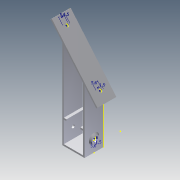
# Autodesk Inventor part: carousel_mount_bracket
Saved by Autodesk Inventor 2011 (Build 150239000, 239)
## iProperties
Created: 2012-12-04
Part Number: carousel_mount_bracket
Document SubType Name: Modeling
Designer: Administrator
Density: 1 g/cm^3
Author: Administrator
Autodesk Inventor part; units mm, degrees
ref_plane "YZ Plane" through (0, 0, 0) normal (1, 0, 0) x (0, 1, 0)
ref_plane "XZ Plane" through (0, 0, 0) normal (0, 1, 0) x (-1, 0, 0)
sketch "Sketch1" plane through (0, 0, 0) normal (0, 0, 1) x (1, 0, 0)
  line L0 (-12.4, 10.5) -> (12.4, 10.5)
  line L1 (12.4, 10.5) -> (12.4, -10.5)
  line L2 (12.4, -10.5) -> (-12.4, -10.5)
  line L3 (-12.4, -10.5) -> (-12.4, 10.5)
  point P0 (0, 0)
  point P1 (-12.4, 0)
  point P2 (0, 10.5)
  dimension "d0" = 24.8
  dimension "d1" = 21
  constraints: 8 end point, 2 midpoint, 2 parallel, 1 horizontal, 1 horizontal alignment, 1 perpendicular, 1 vertical alignment
  measures "d0" distance of L0.start L0.end
  measures "d1" distance between parallel lines of L2 L0
extrude "Extrusion1" add sketch "Sketch1" along normal blind 1.75
ref_plane "Work Plane1" through (0, 0, 84.25) normal (0, 0, 1) x (1, 0, 0)
sketch "Sketch3" plane through (0, 0, 84.25) normal (0, 0, 1) x (1, 0, 0)
  line L0 (0, 9.7015) -> (0, -9.7015) construction
  point P0 (0, 0)
  point P1 (0, 0)
  constraints: 2 end point, 1 coincident, 1 midpoint, 1 vertical
ref_plane "Work Plane2" through (0, 9.7015, 84.25) normal (0.7660444, 0, 0.6427876) x (0, -1, 0)
sketch "Sketch2" plane through (0, 0, 1.75) normal (0, 0, 1) x (1, 0, 0)
  line L0 (12.4, 10.5) -> (12.4, -10.5) projected
  line L1 (-12.4, 10.5) -> (12.4, 10.5) projected
  line L2 (12.4, -10.5) -> (-12.4, -10.5) projected
  line L3 (-12.4, 10.5) -> (-10.65, 10.5)
  line L4 (-10.65, 10.5) -> (-10.65, -10.5)
  line L5 (-10.65, -10.5) -> (-12.4, -10.5)
  line L6 (-12.4, -10.5) -> (-12.4, 10.5)
  line L7 (12.4, -10.5) -> (10.65, -10.5)
  line L8 (10.65, -10.5) -> (10.65, 10.5)
  line L9 (10.65, 10.5) -> (12.4, 10.5)
  line L10 (12.4, 10.5) -> (12.4, -10.5)
  point P0 (0, 0)
  dimension "d4" = 1.75
  dimension "d5" = 1.75
  constraints: 16 end point, 4 parallel, 2 horizontal, 2 perpendicular, 2 point on line
  measures "d4" distance of L1.start L3.end
  measures "d5" distance between parallel lines of L0 L8
extrude "Extrusion2" add sketch "Sketch2" along normal up to surface contours L0 L2 L8 L1 | L4 L2 L6 L1 surface through (0, 9.7015, 84.25) normal (0.7660444, 0, 0.6427876)
sketch "Sketch4" plane through (-12.4, -10.5, 0) normal (0, -1, 0) x (1, 0, 0)
  line L0 (1.75, 96.9422) -> (0, 99.0277) projected
  line L1 (24.8, 69.4723) -> (23.05, 71.5578) projected
  line L2 (23.05, 1.75) -> (23.05, 71.5578) projected
  line L3 (23.05, 71.5578) -> (23.05, 74.2803)
  line L4 (23.05, 74.2803) -> (39.014, 55.2552)
  line L5 (39.014, 55.2552) -> (37.6734, 54.1303)
  line L6 (37.6734, 54.1303) -> (24.8, 69.4723)
  line L7 (0, 99.0277) -> (-12.8734, 114.3697)
  line L8 (-12.8734, 114.3697) -> (-11.5328, 115.4946)
  line L9 (-11.5328, 115.4946) -> (1.75, 99.6647)
  line L10 (1.75, 99.6647) -> (1.75, 96.9422)
  line L11 (24.8, 0) -> (24.8, 69.4723) projected
  line L12 (23.05, 71.5578) -> (23.05, 74.2803)
  line L13 (23.05, 74.2803) -> (1.75, 99.6647)
  line L14 (1.75, 99.6647) -> (1.75, 96.9422)
  line L15 (1.75, 96.9422) -> (23.05, 71.5578)
  point P0 (12.4, 0)
  dimension "d10" = 1.75
  dimension "d11" = 22.75
  dimension "d12" = 1.75
  dimension "d13" = 22.75
  constraints: 24 end point, 4 parallel, 4 perpendicular, 2 collinear
  measures "d10" distance of L4.end L5.end
  measures "d11" distance from line of L5 L1.end
  measures "d12" distance of L7.end L8.end
  measures "d13" distance from line of L8 L0.start
extrude "Extrusion3" add sketch "Sketch4" against normal up to surface (21 mm away)
sketch "Sketch5" plane through (-10.65, -10.5, 1.75) normal (1, 0, 0) x (0, 0, -1)
  line L0 (0, 0) -> (-95.1922, 0) projected
  line L1 (0, 21) -> (-23.3, 21)
  line L2 (-23.3, 21) -> (-23.3, 0)
  line L3 (-23.3, 0) -> (0, 0)
  line L4 (0, 0) -> (0, 21)
  circle A0 centre (-11.65, 10.5) radius 1.7
  point P0 (-97.7359, 0)
  point P1 (1.75, 10.5)
  dimension "d16" = 23.3
  dimension "d17" = 3.4
  constraints: 8 end point, 2 parallel, 1 centre point, 1 horizontal, 1 perpendicular, 1 point on line
  measures "d16" distance of L1.start L1.end
  measures "d17" diameter of A0
extrude "Extrusion4" cut sketch "Sketch5" against normal up to surface (1.75 mm away) contours A0
mirror "Mirror1" about plane through (0, 0, 0) normal (1, 0, 0) of "Extrusion4"
sketch "Sketch8" plane through (-23.9328, -10.5, 115.4946) normal (0.7660444, 0, 0.6427876) x (0.6427876, 0, -0.7660444)
  line L0 (0, 0) -> (0, 21) projected
  line L1 (78.6369, 0) -> (78.6369, 21) projected
  circle A0 centre (10.5, 10.5) radius 1.7
  circle A1 centre (68.1369, 10.5) radius 1.7
  point P0 (103.8577, 10.5)
  point P1 (0, 10.5)
  point P2 (78.6369, 10.5)
  dimension "d25" = 3.4
  dimension "d26" = 3.4
  dimension "d27" = 10.5
  dimension "d28" = 10.5
  constraints: 2 centre point, 2 horizontal alignment, 2 midpoint
  measures "d25" diameter of A0
  measures "d26" diameter of A1
  measures "d27" distance from line of L0 A0.centre
  measures "d28" distance from line of L1 A1.centre
extrude "Extrusion6" cut sketch "Sketch8" against normal up to surface (1.75 mm away)
sketch "Sketch9" plane through (-12.4, -10.5, 99.0277) normal (-0.7660444, 0, -0.6427876) x (-0.6427876, 0, 0.7660444)
  circle A0 centre (9.5275, 10.5) radius 1.7 projected
  line L0 (20.0275, 21) -> (0, 21) projected
  circle A1 centre (9.5275, 10.5) radius 4.3
  line L1 (11.1441, 7.7) -> (7.9109, 7.7)
  line L2 (7.9109, 7.7) -> (6.2943, 10.5)
  line L3 (6.2943, 10.5) -> (7.9109, 13.3)
  line L4 (7.9109, 13.3) -> (11.1441, 13.3)
  line L5 (11.1441, 13.3) -> (12.7606, 10.5)
  line L6 (12.7606, 10.5) -> (11.1441, 7.7)
  circle A2 centre (-48.1094, 10.5) radius 1.7 projected
  line L7 (-38.582, 21) -> (-58.6094, 21) projected
  circle A3 centre (-48.1094, 10.5) radius 4.3
  line L8 (-46.4929, 7.7) -> (-49.726, 7.7)
  line L9 (-49.726, 7.7) -> (-51.3426, 10.5)
  line L10 (-51.3426, 10.5) -> (-49.726, 13.3)
  line L11 (-49.726, 13.3) -> (-46.4929, 13.3)
  line L12 (-46.4929, 13.3) -> (-44.8763, 10.5)
  line L13 (-44.8763, 10.5) -> (-46.4929, 7.7)
  point P0 (-83.8302, 10.5)
  dimension "d31" = 5.6
  dimension "d32" = 1.5
  dimension "d38" = 5.6
  dimension "d39" = 1.5
  constraints: 24 end point, 4 coincident, 2 centre point, 2 parallel, 26 other
  measures "d31" distance between parallel lines of L4 L1
  measures "d32" distance edge to line of A1 L4
  measures "d38" distance between parallel lines of L8 L11
  measures "d39" distance edge to line of A3 L11
extrude "Extrusion7" cut sketch "Sketch9" against normal blind 0.75 contours L1 L2 L3 L4 L5 L6
extrude "Extrusion8" add sketch "Sketch9" along normal blind 1.55 contours A1
draft "FaceDraft1" angle 45 pull direction (-0.7660444, 0, -0.6427876) faces at (-22.0708, -0.346, 108.9453) fixed edges at (-16.9475, 0, 102.0359)
extrude "Extrusion9" cut sketch "Sketch9" against normal blind 0.75 contours L8 L9 L10 L11 L12 L13
extrude "Extrusion10" add sketch "Sketch9" along normal blind 1.55 contours A3
draft "FaceDraft2" angle 45 pull direction (-0.7660444, 0, -0.6427876) faces at (15.0044, -0.6898, 64.7609) fixed edges at (20.1008, 0, 57.8835)
sketch "Sketch10" plane through (12.4, -10.5, 0) normal (1, 0, 0) x (0, 0, -1)
  circle A0 centre (-13.4, 10.5) radius 1.7 projected
  line L0 (0, 21) -> (-69.4723, 21) projected
  circle A1 centre (-13.4, 10.5) radius 4.3
  line L1 (-11.7834, 7.7) -> (-15.0166, 7.7)
  line L2 (-15.0166, 7.7) -> (-16.6332, 10.5)
  line L3 (-16.6332, 10.5) -> (-15.0166, 13.3)
  line L4 (-15.0166, 13.3) -> (-11.7834, 13.3)
  line L5 (-11.7834, 13.3) -> (-10.1668, 10.5)
  line L6 (-10.1668, 10.5) -> (-11.7834, 7.7)
  point P0 (0, 10.5)
  dimension "d45" = 5.6
  dimension "d46" = 1.5
  constraints: 12 end point, 2 coincident, 1 centre point, 1 parallel, 13 other
  measures "d45" distance between parallel lines of L1 L4
  measures "d46" distance edge to line of A1 L4
extrude "Extrusion11" cut sketch "Sketch10" against normal blind 0.75 contours L1 L2 L3 L4 L5 L6
extrude "Extrusion12" add sketch "Sketch10" along normal blind 1.55 contours A1
draft "FaceDraft3" angle 45 pull direction (1, 0, 0) faces at (12.9167, -0.6898, 9.1557) fixed edges at (13.95, 0, 17.7)
sketch "Sketch11" plane through (-10.65, -10.5, 1.75) normal (1, 0, 0) x (0, 0, -1)
  line L0 (0, 0) -> (-95.1922, 0) projected
  line L1 (0, 21) -> (0, 0) projected
  line L2 (0, 21) -> (-95.1922, 21) projected
  line L3 (-25.35, 21) -> (-23.6, 21)
  line L4 (-23.6, 21) -> (-23.6, 0)
  line L5 (-23.6, 0) -> (-25.35, 0)
  line L6 (-25.35, 0) -> (-25.35, 21)
  point P0 (1.75, 10.5)
  dimension "d52" = 1.75
  dimension "d53" = 23.6
  constraints: 8 end point, 2 parallel, 2 point on line, 1 horizontal, 1 perpendicular
  measures "d52" distance between parallel lines of L4 L6
  measures "d53" distance between parallel lines of L4 L1
extrude "Extrusion13" add sketch "Sketch11" along normal blind 3 contours L0 L6 L2 L4
mirror "Mirror2" about plane through (0, 0, 0) normal (1, 0, 0) of "Extrusion13"
equation "\"d4\" = d5"
equation "\"d12\" = d10"
equation "\"d26\" = d25"
equation "\"d28\" = d27"
body "Solid1"
